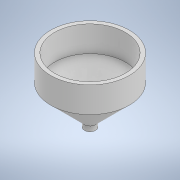
# Autodesk Inventor part: seeder
Saved by Autodesk Inventor 2020 (Build 240168000, 168)
## iProperties
Created: 2020-03-05
Part Number: seeder
Material: Generic
Document SubType Name: Modeling
Designer: Aryan
Density: 1 g/cm^3
Appearance: Default
Author: Aryan
Autodesk Inventor part; units mm, degrees
ref_plane "YZ Plane" through (0, 0, 0) normal (1, 0, 0) x (0, 1, 0)
ref_plane "XZ Plane" through (0, 0, 0) normal (0, 1, 0) x (-1, 0, 0)
ref_plane "XY Plane" through (0, 0, 0) normal (0, 0, 1) x (1, 0, 0)
sketch "Sketch1" plane through (0, 0, 0) normal (1, 0, 0) x (0, 1, 0)
  line L0 (0, 0) -> (50, 0)
  line L1 (50, 0) -> (50, 30.5)
  line L2 (50, 30.5) -> (30, 30.5)
  line L3 (30, 30.5) -> (3.837, 4.337)
  line L4 (3.837, 4.337) -> (0, 4.337)
  line L5 (0, 4.337) -> (0, 1.337)
  line L6 (0, 1.337) -> (3.837, 1.337)
  line L7 (3.837, 1.337) -> (30, 27.5)
  line L8 (30, 27.5) -> (50, 27.5)
  dimension "d0" = 50
  dimension "d1" = 30.5
  dimension "d2" = 20
  dimension "d3" = 90
  dimension "d4" = 37
  dimension "d5" = 135
  dimension "d6" = 3
  constraints: 18 end point, 5 perpendicular, 2 parallel, 1 horizontal, 1 point on line
  measures "d0" distance of L0.start L0.end
  measures "d1" distance of L0.end L1.end
  measures "d2" distance of L1.end L2.end
  measures "d3" angle of L2 L1
  measures "d4" distance of L2.end L3.end
  measures "d5" angle of L3 L2
  measures "d6" distance of L4.end L5.end
revolve "Revolution1" add sketch "Sketch1" angle 360 about axis through (0, 0, 0) along (0, 1, 0)
body "Solid1"
